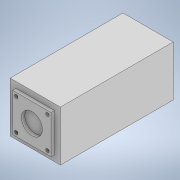
# Autodesk Inventor part: toppmt
Saved by Autodesk Inventor 2022.2 (Build 262287030, 287C)
## iProperties
Created: 2022-02-04
Part Number: toppmt
Material: Generic
Document SubType Name: Modeling
Designer: Tapendra
Density: 1 g/cm^3
Appearance: Default
Author: Tapendra
Autodesk Inventor part; units mm, degrees
ref_plane "YZ Plane" through (0, 0, 0) normal (1, 0, 0) x (0, 1, 0)
ref_plane "XZ Plane" through (0, 0, 0) normal (0, 1, 0) x (-1, 0, 0)
ref_plane "XY Plane" through (0, 0, 0) normal (0, 0, 1) x (1, 0, 0)
sketch "Sketch1" plane through (0, 0, 0) normal (0, 0, 1) x (1, 0, 0)
  line L0 (-11.25, 11.25) -> (11.25, 11.25)
  line L1 (11.25, 11.25) -> (11.25, -11.25)
  line L2 (11.25, -11.25) -> (-11.25, -11.25)
  line L3 (-11.25, -11.25) -> (-11.25, 11.25)
  line L4 (-11.25, 11.25) -> (11.25, -11.25) construction
  line L5 (11.25, 11.25) -> (-11.25, -11.25) construction
  point P0 (0, 0)
  dimension "d0" = 22.5
  dimension "d1" = 22.5
  constraints: 12 end point, 2 midpoint, 2 parallel, 1 horizontal, 1 perpendicular
  measures "d0" distance of L0.start L0.end
  measures "d1" distance of L0.end L1.end
extrude "Extrusion1" add sketch "Sketch1" along normal mid plane 50.5
sketch "Sketch8" plane through (0, 0, 25.25) normal (0, 0, 1) x (1, 0, 0)
  line L0 (-8.6, 8.6) -> (8.6, 8.6)
  line L1 (8.6, 8.6) -> (8.6, -8.6)
  line L2 (8.6, -8.6) -> (-8.6, -8.6)
  line L3 (-8.6, -8.6) -> (-8.6, 8.6)
  line L4 (-8.6, 8.6) -> (8.6, -8.6) construction
  line L5 (8.6, 8.6) -> (-8.6, -8.6) construction
  circle A0 centre (0, 0) radius 4.715
  dimension "d41" = 17.2
  dimension "d42" = 17.2
  dimension "d43" = 9.43
  constraints: 12 end point, 2 midpoint, 2 parallel, 1 centre point, 1 coincident, 1 horizontal, 1 perpendicular
  measures "d41" distance of L0.start L0.end
  measures "d42" distance of L0.end L1.end
  measures "d43" diameter of A0
extrude "Extrusion4" add sketch "Sketch8" along normal blind 1.5
sketch "Sketch9" plane through (0, 0, 26.75) normal (0, 0, 1) x (1, 0, 0)
  line L0 (-8.6, -8.6) -> (8.6, -8.6) projected
  line L1 (8.6, -8.6) -> (8.6, 8.6) projected
  line L2 (8.6, 8.6) -> (-8.6, 8.6) projected
  line L3 (-8.6, 8.6) -> (-8.6, -8.6) projected
  circle A0 centre (0, 0) radius 4.715 projected
  line L4 (-8.6, -8.6) -> (8.6, -8.6) projected
  line L5 (8.6, -8.6) -> (8.6, 8.6) projected
  line L6 (8.6, 8.6) -> (-8.6, 8.6) projected
  line L7 (-8.6, 8.6) -> (-8.6, -8.6) projected
  circle A1 centre (0, 0) radius 4.715 projected
  point P0 (-7, 7)
  point P1 (7, 7)
  point P2 (-7, -7)
  point P3 (7, -7)
  dimension "d48" = 14
  dimension "d51" = 14
  dimension "d54" = 7
  dimension "d55" = 7
  constraints: 1 horizontal, 1 vertical, 3 other
  measures "d48" distance of point (-7, 7) point (7, 7)
  measures "d51" distance of point (-7, 7) point (-7, -7)
  measures "d54" horizontal distance of point (-7, 7) point (0, 0)
  measures "d55" horizontal distance of point (-7, 7) point (0, 0)
hole "Hole3" at (-7, 7, 26.75) at (7, 7, 26.75) at (-7, -7, 26.75) at (7, -7, 26.75) direction (0, 0, -1) diameter 1.567 depth 3 tip angle 118 thread size "M2x0.4" class "6H" standard "ANSI Metric M Profile"
equation "\"d42\" = d41"
body "Solid1"
